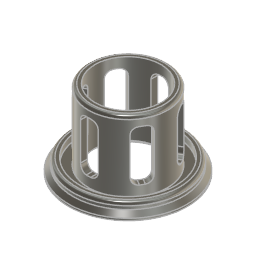
propogation_basket_open_bottom (Autodesk Fusion 360 design; units mm, degrees)
Autodesk Fusion 360 part; units mm, degrees
sketch "insert_base" plane through (0, 0, 0) normal (0, 0, 1) x (1, 0, 0)
  circle A0 centre (0, 0) radius 25
  circle A1 centre (0, 0) radius 28
  circle A2 centre (0, 0) radius 22
  circle A3 centre (0, 0) radius 27
  dimension "d22" = 50
  dimension "d23" = 56
  dimension "d24" = 44
  dimension "d109" = 54
  constraint coincident A0.centre A1.centre
  constraint concentric A0 A2
  measures "d22" diameter of A0
  measures "d23" diameter of A1
  measures "d24" diameter of A2
  measures "d109" diameter of A3
extrude "Extrude4" add sketch "insert_base" along normal blind 6 contours A0 makes body 1
extrude "Extrude5" add sketch "insert_base" along normal blind 3 contours A1 | A3 bodies 1
chamfer "Chamfer2" distance 3 angle 45 1 edges at (-26.1052, -10.1252, 3) on bodies 1
sketch "basket_base" plane through (0, 0, 0) normal (0, 0, 1) x (1, 0, 0)
  circle A0 centre (0, 0) radius 25
  circle A1 centre (0, 0) radius 15
  circle A2 centre (0, 0) radius 18
  dimension "d30" = 50
  dimension "d31" = 30
  dimension "d32" = 36
  constraint coincident A0.centre A1.centre
  constraint concentric A0 A2
  measures "d30" diameter of A0
  measures "d31" diameter of A1
  measures "d32" diameter of A2
copy_body "CopyPasteBodies1" bodies 1 makes body 2
extrude "Extrude6" add sketch "basket_base" along normal blind 3 contours A0 bodies 2
extrude "Extrude7" add sketch "basket_base" along normal blind 35 contours A2 bodies 2
fillet "Fillet3" radius 1.5 1 edges at (-16.7819, -6.5091, 35) on bodies 2
fillet "Fillet4" radius 1.5 1 edges at (-23.3082, -9.0404, 6) on bodies 2
fillet "Fillet5" radius 1.5 1 edges at (-23.3082, -9.0404, 6) on bodies 1
chamfer "Chamfer3" distance 2 angle 45 1 edges at (-13.9849, 5.4242, 0) on bodies 2
sketch "basket_cutout" plane through (0, 0, 0) normal (0, 1, 0) x (1, 0, 0)
  line L0 (0, 0) -> (0, -0.8242)
  line L1 (0, 0) -> (4, 0)
  line L2 (4, 0) -> (-4, 0)
  line L3 (-4, -10.5) -> (-4, -27.5)
  line L4 (-1, -30.5) -> (1, -30.5)
  line L5 (4, -27.5) -> (4, -10.5)
  line L6 (4, 0) -> (-4, 0)
  line L7 (-4, 0) -> (-4, -7.5)
  line L8 (-1, -7.5) -> (1, -7.5)
  line L9 (4, -7.5) -> (4, 0)
  arc A0 (1, -30.5) -> (4, -27.5) centre (1, -27.5) ccw
  arc A1 (-4, -27.5) -> (-1, -30.5) centre (-1, -27.5) ccw
  arc A2 (4, -10.5) -> (1, -7.5) centre (1, -10.5) ccw
  arc A3 (-1, -7.5) -> (-4, -10.5) centre (-1, -10.5) ccw
  point P0 (4, -30.5)
  dimension "d93" = 4
  dimension "d94" = 8
  dimension "d95" = 30.5
  dimension "d96" = 7.5
  dimension "d98" = 3
  dimension "d99" = 3
  dimension "d100" = 3
  dimension "d101" = 3
  constraint coincident L0.start L1.start
  constraint vertical L0
  constraint perpendicular L0 L1
  constraint horizontal L2
  constraint vertical L3
  constraint horizontal L4
  constraint vertical L5
  constraint horizontal L6
  constraint vertical L7
  constraint horizontal L8
  constraint vertical L9
  constraint coincident P0 L4
  constraint coincident P0 L5
  constraint tangent L4 A0
  constraint tangent L5 A0
  constraint tangent L4 A1
  constraint tangent L3 A1
  constraint coincident L1.end L5
  constraint coincident L9.start L8
  constraint tangent L5 A2
  constraint tangent L8 A2
  constraint coincident L7.end L8
  constraint coincident L2.end L3
  constraint tangent L8 A3
  constraint tangent L3 A3
  measures "d93" distance of L0.start L1.end
  measures "d94" distance of L1.end L2.end
  measures "d95" distance of L1.end P0
  measures "d96" distance of L1.end L9.start
  measures "d98" radius of A0
  measures "d99" radius of A1
  measures "d100" radius of A2
  measures "d101" radius of A3
extrude "Extrude12" cut sketch "basket_cutout" along normal blind 18 bodies 2
pattern_circular "C-Pattern4" count 6 over 360 about axis through (0, 0, 1.75) along (0, 0, 1) of "Extrude12"
extrude "Extrude13" cut sketch "insert_base" along normal blind 6 contours A1 bodies 2
hidden bodies 1
equation "wall_thickness = 3 mm" comment "Thickness off the walls of the insert, the walls of the basket, the flat top, etc."
equation "_insert_outer_diameter = 50 mm" comment "Do not edit."
equation "d22 = _insert_outer_diameter"
equation "d23 = _insert_outer_diameter + ( 2 * wall_thickness )"
equation "d24 = _insert_outer_diameter - ( 2 * wall_thickness )"
equation "d25 = wall_thickness * 2"
equation "d27 = wall_thickness"
equation "d29 = wall_thickness"
equation "d30 = _insert_outer_diameter"
equation "d31 = basket_inner_diameter"
equation "d32 = basket_inner_diameter + ( wall_thickness * 2 )"
equation "d33 = wall_thickness"
equation "d35 = basket_length"
equation "d63 = basket_opening_chamfer"
equation "basket_length = 35 mm" comment "Max length of the basket."
equation "basket_cutout_num = 6" comment "Number of holes in the basket."
equation "basket_cutout_width = 8 mm" comment "Width of the holes in the basket."
equation "basket_cutout_distance_from_edge = 4.5 mm" comment "Distance from the bottom of the basket hole cutout, and the floor geometry, also distance down from max length of the basket."
equation "d93 = basket_cutout_width / 2"
equation "d94 = basket_cutout_width"
equation "d95 = basket_length - basket_cutout_distance_from_edge"
equation "d96 = basket_cutout_distance_from_edge + wall_thickness"
equation "d98 = ( basket_cutout_width / 2 ) - 1 mm"
equation "d99 = ( basket_cutout_width / 2 ) - 1 mm"
equation "d100 = ( basket_cutout_width / 2 ) - 1 mm"
equation "d101 = ( basket_cutout_width / 2 ) - 1 mm"
equation "basket_inner_diameter = 30 mm" comment "Width of the basket, bigger for wider basket, limited to insert_outer_diameter."
equation "d103 = basket_inner_diameter / 2 + wall_thickness"
equation "d105 = basket_cutout_num"
equation "insert_overhang_edge_cutoff = 1 mm" comment "Blunt the insert overhang that fits into the adapter, by cutting off some of the edge."
equation "basket_opening_chamfer = 2 mm" comment "Chamfer the opening of the basket, to soften the edge where cuttings are inserted."
equation "d109 = _insert_outer_diameter + ( 2 * wall_thickness ) - ( 2 * insert_overhang_edge_cutoff )"
equation "d110 = wall_thickness * 2"
named bodies: "test_insert", "insert", "progration_basket_30m_closed"
